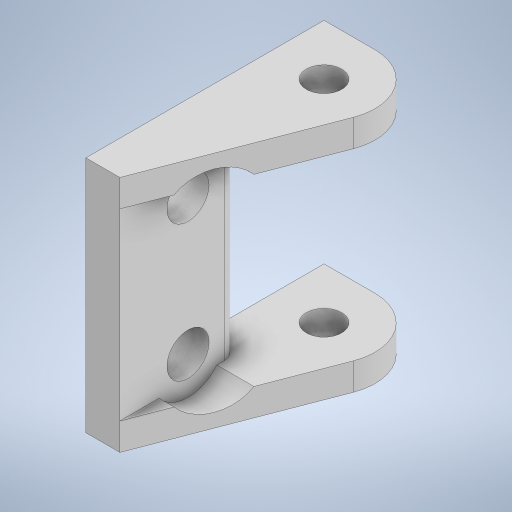
# Autodesk Inventor part: IdlerPulley Holder
Saved by Autodesk Inventor 2023 (Build 270158000, 158)
## iProperties
Created: 2023-04-27
Part Number: IdlerPulley Holder
Material: Generic
Document SubType Name: Modeling
Designer: ethan
Density: 1 g/cm^3
Appearance: Default
Author: ethan
Autodesk Inventor part; units mm, degrees
ref_plane "YZ Plane" through (0, 0, 0) normal (1, 0, 0) x (0, 1, 0)
ref_plane "XZ Plane" through (0, 0, 0) normal (0, 1, 0) x (-1, 0, 0)
ref_plane "XY Plane" through (0, 0, 0) normal (0, 0, 1) x (1, 0, 0)
sketch "Sketch1" plane through (0, 0, 0) normal (0, 1, 0) x (-1, 0, 0)
  line L0 (0, 0) -> (-20, 0) construction
  line L1 (-20, 0) -> (-20, -20) construction
  line L2 (-20, -20) -> (0, -20) construction
  line L3 (0, -20) -> (0, 0) construction
  circle A0 centre (-27.5, -27.5) radius 2.6
  circle A1 centre (-27.5, -27.5) radius 9 construction
  line L4 (-20, 0) -> (-25, 0)
  line L5 (-25, 0) -> (-25, -20)
  line L6 (-20, -20) -> (-20, 0)
  arc A2 (-27.5, -20) -> (-27.5, -35) centre (-27.5, -27.5) ccw
  line L7 (-27.5, -35) -> (-20, -35)
  line L8 (-20, -20) -> (-20, -35)
  arc A3 (-27.5, -35) -> (-27.5, -20) centre (-27.5, -27.5) ccw construction
  line L9 (-27.5, -20) -> (-25, -20)
  circle A4 centre (-27.5, -27.5) radius 11
  line L10 (-34.504, -24.8178) -> (-25, 0)
  point P0 (-20, -19.4533)
  point P1 (-31.6263, -17.3032)
  dimension "d0" = 20
  dimension "d1" = 20
  dimension "d4" = 5.2
  dimension "d11" = 7.5
  dimension "d12" = 18
  dimension "d14" = 7.5
  dimension "d15" = 5
  dimension "d16" = 15
  dimension "d34" = 2
  dimension "d36" = 0
  constraints: 23 end point, 6 point on circle, 5 centre point, 4 horizontal, 3 coincident, 3 parallel, 3 tangent, 2 perpendicular, 1 collinear, 1 point on line
  measures "d0" distance of L2.end L1.end
  measures "d1" distance of L1.end L0.end
  measures "d4" diameter of A0
  measures "d11" horizontal distance of L1.end A0.centre
  measures "d12" diameter of A1
  measures "d14" horizontal distance of A1.centre L1.end
  measures "d15" distance of L1.end L5.end
  measures "d16" diameter of A2
  measures "d34" radial gap between concentric circles of A1 A4
  measures "d36" distance from line of L4 L10.end
extrude "Extrusion1" add sketch "Sketch1" along normal mid plane 35 contours L6 A4 L5 L4 | L6 L8 L7 A2 L9 L5 A4
extrude "Extrusion4" cut sketch "Sketch1" along normal mid plane 27 contours A4 L10 A2 L7 L8 L6 | L6 L8 L7 A2 L9 L5 A4 | L5 L9 A2 L10 A4
sketch "Sketch3" plane through (25, -17.5, 0) normal (1, 0, 0) x (0, 0, -1)
  line L0 (35, 35) -> (0, 35) construction
  line L1 (10, 34.6833) -> (10, 0) construction
  circle A0 centre (10, 27.5) radius 3.1
  circle A1 centre (10, 7.5) radius 3.1
  circle A2 centre (10, 27.5) radius 5.5
  circle A3 centre (10, 7.5) radius 5.5
  line L2 (20, 0) -> (0, 0) projected
  line L3 (0, 0) -> (0, 35) projected
  point P0 (20, 35)
  point P1 (16.4634, 0)
  dimension "d22" = 6.2
  dimension "d23" = 6.2
  dimension "d24" = 7.5
  dimension "d41" = 11
  dimension "d42" = 11
  dimension "d43" = 7.5
  dimension "d50" = 10
  constraints: 4 centre point, 2 coincident, 2 end point, 2 point on line, 1 vertical
  measures "d22" diameter of A0
  measures "d23" diameter of A1
  measures "d24" distance from line of L0 A0.centre
  measures "d41" diameter of A2
  measures "d42" diameter of A3
  measures "d43" distance from line of L2 A1.centre
  measures "d50" distance between parallel lines of L3 L1
extrude "Extrusion3" cut sketch "Sketch3" against normal up to surface (5 mm away) contours A0 | A1
extrude "Extrusion5" add sketch "Sketch1" along normal mid plane 35 contours L5 A4 L10 | L5 L9 A2 L10 A4
extrude "Extrusion6" cut sketch "Sketch1" along normal mid plane 27 contours L5 A4 L10 | L5 L9 A2 L10 A4
extrude "Extrusion7" cut sketch "Sketch3" along normal up to next
fillet "Fillet3" radius 2 1 edges at (25, 0, -16.7879)
body "Solid1"
